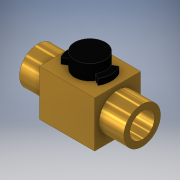
# Autodesk Inventor part: BBBB
Saved by Autodesk Inventor 2016 SP2 (Build 200236200, 236)
## iProperties
Created: 2017-03-30
Part Number: BBBB
Material: Brass
Document SubType Name: Modeling
Designer: smiku
Mass: 90.5814 g
Surface Area: 61.4235 cm^2
Volume: 10.6692 cm^3
Density: 8.49 g/cm^3
Appearance: Brass - Polished
Author: smiku
Autodesk Inventor part; units mm, degrees
ref_plane "YZ Plane" through (0, 0, 0) normal (1, 0, 0) x (0, 1, 0)
ref_plane "XZ Plane" through (0, 0, 0) normal (0, 1, 0) x (-1, 0, 0)
ref_plane "XY Plane" through (0, 0, 0) normal (0, 0, 1) x (1, 0, 0)
sketch "Sketch1" plane through (0, 0, 0) normal (1, 0, 0) x (0, 1, 0)
  line L0 (-9.525, 9.525) -> (9.525, 9.525)
  line L1 (9.525, 9.525) -> (9.525, -9.525)
  line L2 (9.525, -9.525) -> (-9.525, -9.525)
  line L3 (-9.525, -9.525) -> (-9.525, 9.525)
  line L4 (-9.525, 9.525) -> (9.525, -9.525) construction
  line L5 (9.525, 9.525) -> (-9.525, -9.525) construction
  circle A0 centre (0, 0) radius 5.08
  circle A1 centre (0, 0) radius 7.62
  dimension "d0" = 19.05
  dimension "d1" = 19.05
  dimension "d2" = 10.16
  dimension "d5" = 15.24
  constraints: 12 end point, 4 midpoint, 2 centre point, 2 parallel, 1 coincident, 1 horizontal, 1 perpendicular
  measures "d0" distance of L1.end L2.end
  measures "d1" distance of L0.end L1.end
  measures "d2" diameter of A0
  measures "d5" diameter of A1
extrude "Extrusion1" add sketch "Sketch1" along normal mid plane 22.86 contours L0 L1 L2 L3 | A1
extrude "Extrusion2" add sketch "Sketch1" along normal mid plane 43.18 contours A1
sketch "Sketch2" plane through (-11.43, -9.525, -9.525) normal (0, -1, 0) x (1, 0, 0)
  circle A0 centre (11.43, 9.525) radius 6.35
  dimension "d8" = 12.7
  constraints: 1 centre point, 1 coincident
  measures "d8" diameter of A0
extrude "Extrusion3" cut sketch "Sketch2" against normal through all
sketch "Sketch3" plane through (-11.43, -9.525, -9.525) normal (0, -1, 0) x (1, 0, 0)
  circle A0 centre (11.43, 9.525) radius 6.35 projected
extrude "Extrusion4" add sketch "Sketch3" along normal blind 2.54 separate body
sketch "Sketch4" plane through (0, -9.525, 0) normal (0, 1, 0) x (1, 0, 0)
  circle A0 centre (0, 0) radius 6.35 projected
extrude "Extrusion5" add sketch "Sketch4" along normal blind 25.4 bodies 2
sketch "Sketch5" plane through (-11.43, 9.525, 9.525) normal (0, 1, 0) x (1, 0, 0)
  circle A0 centre (11.43, 9.525) radius 6.35 construction
  circle A1 centre (11.43, 9.525) radius 8.89 construction
  line L0 (2.54, 9.525) -> (20.32, 9.525) construction
  line L1 (3.731, 5.08) -> (19.129, 13.97) construction
  line L2 (3.731, 13.97) -> (19.129, 5.08) construction
  circle A2 centre (11.43, 9.525) radius 6.35 construction
  arc A3 (16.9293, 6.35) -> (16.9293, 12.7) centre (11.43, 9.525) ccw
  arc A4 (19.129, 5.08) -> (19.129, 13.97) centre (11.43, 9.525) ccw
  arc A5 (5.9307, 12.7) -> (5.9307, 6.35) centre (11.43, 9.525) ccw
  arc A6 (3.731, 13.97) -> (3.731, 5.08) centre (11.43, 9.525) ccw
  line L3 (5.9307, 12.7) -> (3.731, 13.97)
  line L4 (5.9307, 6.35) -> (3.731, 5.08)
  line L5 (19.129, 13.97) -> (16.9293, 12.7)
  line L6 (16.9293, 6.35) -> (19.129, 5.08)
  dimension "d15" = 17.78
  dimension "d16" = 30
  dimension "d17" = 30
  constraints: 16 point on circle, 14 end point, 5 centre point, 5 coincident, 3 collinear, 2 line through centre, 2 point on line, 1 horizontal
  measures "d15" diameter of A1
  measures "d16" angle of L0 L1
  measures "d17" angle of L0 L2
extrude "Extrusion6" add sketch "Sketch5" along normal blind 2.54 bodies 2
body "Solid1"
body "Solid2"
